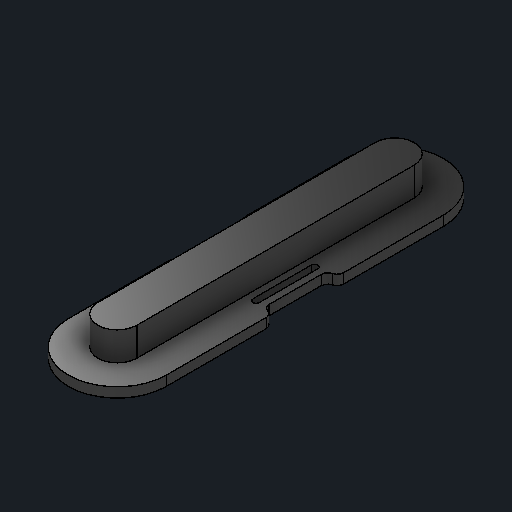
# Autodesk Inventor part: CableWrapCore
Saved by Autodesk Inventor 2026.2 (Build 302298000, 298)
## iProperties
Created: 2026-02-07
Part Number: CableWrapCore
Material: ABS Plastic
Document SubType Name: Modeling
Designer: JoshuaEah
Density: 1.06 g/cm^3
Appearance: Glossy - Black
Author: JoshuaEah
Autodesk Inventor part; units mm, degrees
ref_plane "YZ Plane" through (0, 0, 0) normal (1, 0, 0) x (0, 1, 0)
ref_plane "XZ Plane" through (0, 0, 0) normal (0, 1, 0) x (-1, 0, 0)
sketch "Sketch2" plane through (0, 0, 0) normal (0, 1, 0) x (-1, 0, 0)
  line L0 (0, 0) -> (-30, 0)
  line L1 (-30, 0) -> (-30, -115)
  line L2 (-30, -115) -> (0, -115)
  line L3 (0, -115) -> (0, 0)
  line L4 (-15, -115) -> (-15, 0)
  line L5 (-9, -106) -> (-21, -106)
  line L6 (-21, -106) -> (-21, -9)
  line L7 (-21, -9) -> (-9, -9)
  line L8 (-9, -9) -> (-9, -106)
  line L9 (-9, -106) -> (-21, -9) construction
  line L10 (-21, -106) -> (-9, -9) construction
  line L11 (0, -57.5) -> (-30, -57.5) construction
  line L12 (-5, -67.5) -> (-7, -67.5)
  line L13 (-5, -47.5) -> (-7, -47.5)
  line L14 (-5, -67.5) -> (-5, -47.5)
  line L15 (-7, -47.5) -> (-7, -67.5)
  line L16 (0, -47.5) -> (-3, -47.5)
  line L17 (-3, -47.5) -> (-3, -67.5)
  line L18 (0, -67.5) -> (-3, -67.5)
  point P0 (-15, -57.5)
  dimension "d0" = 30
  dimension "d1" = 115
  dimension "d2" = 12
  dimension "d3" = 9
  dimension "d4" = 9
  dimension "d12" = 2
  dimension "d13" = 20
  dimension "d17" = 2
  dimension "d21" = 20
  dimension "d22" = 2
  constraints: 38 end point, 7 midpoint, 5 parallel, 5 perpendicular, 4 symmetric about line, 3 horizontal, 2 point on line, 1 coincident, 1 vertical
  measures "d0" distance of L2.end L1.end
  measures "d1" distance of L1.end L0.end
  measures "d2" distance of L6.end L7.end
  measures "d3" distance between parallel lines of L3 L8
  measures "d4" distance between parallel lines of L2 L5
  measures "d12" distance of L12.start L12.end
  measures "d13" distance of L12.start L13.start
  measures "d17" distance between parallel lines of L8 L15
  measures "d21" distance of L16.end L17.end
  measures "d22" distance between parallel lines of L14 L17
extrude "Extrusion1" add sketch "Sketch2" against normal blind 3 contours L3 L16 L17 L18 L2 L4 L5 L8 L7 L0 | L4 L7 L6 L5 L2 L1 L0 | L3 L18 L17 L16 | L7 L8 L5 L4 | L4 L5 L6 L7 | L12 L15 L13 L14
extrude "Extrusion2" add sketch "Sketch2" along normal blind 8.75 contours L7 L8 L5 L4 | L4 L5 L6 L7
ref_plane "Work Plane1" through (15, 0, -9) normal (-1, 0, 0) x (0, 0, 1)
fillet "Fillet1" radius 6 4 edges at (21, 4.375, -9) (9, 4.375, -9) (9, 4.375, -106) (21, 4.375, -106)
fillet "Fillet2" radius 15 4 edges at (30, -1.5, 0) (0, -1.5, 0) (0, -1.5, -115) (30, -1.5, -115)
extrude "Extrusion3" cut sketch "Sketch2" against normal through all contours L12 L15 L13 L14
fillet "Fillet3" radius 1 4 edges at (7, -1.5, -67.5) (5, -1.5, -67.5) (5, -1.5, -47.5) (7, -1.5, -47.5)
extrude "Extrusion4" cut sketch "Sketch2" against normal through all contours L3 L18 L17 L16
fillet "Fillet4" radius 2 2 edges at (3, -1.5, -67.5) (3, -1.5, -47.5)
fillet "Fillet5" radius 2 2 edges at (0, -1.5, -67.5) (0, -1.5, -47.5)
mirror "Mirror2" about plane through (15, 0, -9) normal (-1, 0, 0) of "Extrusion3", "Fillet3", "Extrusion4", "Fillet4", "Fillet5"
equation "\"d4\" = d3"
equation "\"d22\" = d17"
equation "\"d9\" = 0.5 * d2"
equation "\"d10\" = 0.5 * d0"
equation "\"d16\" = 0.5 * d12"
body "Solid1"
